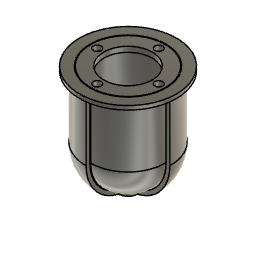
duba alt 2 v2 (Autodesk Fusion 360 design; units mm, degrees)
Autodesk Fusion 360 part; units mm, degrees
sketch "Eskiz1" plane through (0, 0, 0) normal (1, 0, 0) x (0, 1, 0)
  line L0 (-18.5, 0) -> (-28.5, 0)
  line L1 (-18.5, 0) -> (-18.5, -4)
  line L2 (-18.5, -4) -> (-28.5, -4)
  line L3 (-28.5, -4) -> (-28.5, 0)
  line L4 (-28.5, -4) -> (-25.5, -4)
  line L5 (-25.5, -4) -> (-25.5, -50)
  line L6 (-25.5, -50) -> (-28.5, -50)
  line L7 (-28.5, -50) -> (-28.5, -4)
  arc A0 (-28.5, -50) -> (-3.5325, -78.2802) centre (0, -50) ccw
  line L8 (-3.5325, -73.2631) -> (-3.5325, -72.7631)
  line L9 (-3.5325, -72.7631) -> (0, -72.7631)
  line L10 (-3.5325, -73.2631) -> (-3.5325, -75.2541)
  line L11 (-3.5325, -72.7631) -> (-5.5325, -72.7631)
  line L12 (-5.5325, -72.7631) -> (-5.5325, -74.8926)
  line L13 (-5.5325, -72.7631) -> (-5.5325, -70.7631)
  line L14 (-5.5325, -70.7631) -> (0, -70.7631)
  line L15 (0, -72.7631) -> (0, -70.7631)
  arc A1 (-25.5, -50) -> (-5.5325, -74.8926) centre (0, -50) ccw
  line L16 (-3.5325, -75.2541) -> (-3.5325, -78.2802)
  dimension "d2" = 10
  dimension "d3" = 2
  dimension "d4" = 2
  constraint perpendicular L0 L1
  constraint perpendicular L1 L2
  constraint coincident L2 L4.end
  constraint perpendicular L0 L5
  constraint perpendicular L5 L6
  constraint concentric A0 A1
  constraint tangent L5 A1
  constraint perpendicular L8 L9
  constraint coincident L10.end A1
  constraint perpendicular L9 L10
  constraint perpendicular L8 L11
  constraint perpendicular L11 L12
  constraint perpendicular L11 L13
  constraint perpendicular L14 L15
  constraint parallel L10 L16
  measures "d2" distance of L0.start L0.end
  measures "d3" distance of L8.end L11.end
  measures "d4" distance of L11.end L13.end
revolve "Döndür1" add sketch "Eskiz1" angle 110 about axis through (0, 0, 1.75) along (0, 0, 1) makes body 1
pattern_circular "C-Desen1" count 2 over 360 about axis through (0, 0, 1.75) along (0, 0, 1) of bodies 1 makes body 2
sketch "Eskiz2" plane through (0, 0, 0) normal (1, 0, 0) x (0, 1, 0)
  line L0 (3.5325, -72.7631) -> (3.5325, -78.2802)
  arc A0 (3.5325, -78.2802) -> (28.5, -50) centre (0, -50) ccw
  line L1 (28.5, -50) -> (28.5, -4)
  line L2 (28.5, -4) -> (28.5, 0)
  line L3 (28.5, 0) -> (18.5, 0)
  line L4 (18.5, 0) -> (18.5, -4)
  line L5 (18.5, -4) -> (25.5, -4)
  line L6 (25.5, -4) -> (25.5, -50)
  arc A1 (5.5325, -74.8926) -> (25.5, -50) centre (0, -50) ccw
  line L7 (5.5325, -74.8926) -> (5.5325, -70.7631)
  line L8 (5.5325, -70.7631) -> (0, -70.7631)
  line L9 (0, -70.7631) -> (0, -72.7631)
  line L10 (0, -72.7631) -> (3.5325, -72.7631)
  line L11 (5.5325, -74.8926) -> (5.5325, -77.9578)
  constraint coincident A1.start L7.start
  constraint coincident A0 L11.end
  constraint parallel L7 L11
revolve "Döndür2" add sketch "Eskiz2" angle 360 about axis through (0, 0, 1.75) along (0, 0, 1) contours L0 A0 L7 L8 L9 L10 L11 bodies 1 2
sketch "Eskiz3" plane through (0, 0, 0) normal (1, 0, 0) x (0, 1, 0)
  line L0 (5.5325, -74.8926) -> (5.5325, -77.9578)
  arc A0 (5.5325, -77.9578) -> (28.5, -50) centre (0, -50) ccw
  line L1 (28.5, -50) -> (28.5, -4)
  line L2 (28.5, -4) -> (28.5, 0)
  line L3 (28.5, 0) -> (18.5, 0)
  line L4 (18.5, 0) -> (18.5, -4)
  line L5 (18.5, -4) -> (25.5, -4)
  line L6 (25.5, -4) -> (25.5, -50)
  arc A1 (5.5325, -74.8926) -> (25.5, -50) centre (0, -50) ccw
  line L7 (18.5, 0) -> (28.5, 0)
  line L8 (28.5, 0) -> (28.5, -4)
  line L9 (28.5, -4) -> (18.5, -4)
  line L10 (18.5, -4) -> (18.5, 0)
  constraint horizontal L7
  constraint vertical L8
  constraint horizontal L9
  constraint vertical L10
  constraint coincident L1.end L2.start
  constraint coincident L3.end L4.start
revolve "Döndür3" add sketch "Eskiz3" angle 360 about axis through (0, 0, 1.75) along (0, 0, 1) contours L2 L3 L4 L5 L7 L8 L9 L10 bodies 1
sketch "Eskiz4" plane through (0, 0, 0) normal (0, 0, 1) x (-1, 0, 0)
  circle A0 centre (0, 0) radius 18.5
  circle A1 centre (0, 0) radius 28.5
  circle A2 centre (0, 23.5) radius 3
  circle A3 centre (-23.5, 0) radius 3
  circle A4 centre (0, -23.5) radius 3
  circle A5 centre (23.5, 0) radius 3
  dimension "d12" = 6
  dimension "d14" = 360
  measures "d12" diameter of A2
extrude "Ekstrüde Et1" cut sketch "Eskiz4" against normal blind 4 contours A2 | A3 | A4 | A5 bodies 1
sketch "Eskiz5" plane through (0, 0, 0) normal (0, 1, 0) x (1, 0, 0)
  line L0 (29, 0) -> (32, 0)
  line L1 (32, 3) -> (32, 50)
  line L2 (29, 50) -> (29, 0)
  line L3 (0, 82) -> (0, 79)
  arc A0 (32, 50) -> (0, 82) centre (0, 50) ccw
  arc A1 (29, 50) -> (0, 79) centre (0, 50) ccw
  line L4 (32, 0) -> (37, 0)
  line L5 (37, 0) -> (37, 3)
  line L6 (37, 3) -> (32, 3)
  constraint perpendicular L0 L1
  constraint concentric A0 A1
  constraint vertical L3
  constraint horizontal L4
  constraint vertical L5
  constraint horizontal L6
revolve "Döndür4" add sketch "Eskiz5" angle 90 about axis through (0, 0, -82) along (0, 0, 1) separate body makes body 3
pattern_circular "C-Desen2" count 2 over 360 about axis through (0, 0, -82) along (0, 0, 1) of bodies 3 makes body 4
sketch "Eskiz6" plane through (0, 0, 0) normal (-1, 0, 0) x (0, -1, 0)
  line L0 (-29, -50) -> (-29, 0)
  line L1 (-29, 0) -> (-37, 0)
  line L2 (-37, 0) -> (-37, -3)
  line L3 (-37, -3) -> (-32, -3)
  line L4 (-32, -3) -> (-32, -50)
  arc A0 (-32, -50) -> (0, -82) centre (0, -50) ccw
  line L5 (0, -82) -> (0, -79)
  arc A1 (-29, -50) -> (0, -79) centre (0, -50) ccw
  line L6 (0, -79.7) -> (-3, -79.7)
  line L7 (-3, -79.7) -> (-3, -78.5)
  line L8 (-3, -78.5) -> (-3, -78.3)
  line L9 (-3, -78.3) -> (-3, -73.3)
  line L10 (-3, -73.3) -> (0, -73.3)
  line L11 (0, -73.3) -> (0, -79.7)
  dimension "d20" = 5
  constraint coincident L5 L6.start
  constraint perpendicular L5 L6
  constraint perpendicular L6 L7
  constraint parallel L7 L8
  constraint parallel L8 L9
  constraint perpendicular L9 L10
  constraint perpendicular L6 L11
  measures "d20" distance of L8.end L9.end
revolve "Döndür5" add sketch "Eskiz6" angle 360 about axis through (0, 0, -73.3) along (0, 0, -1) contours A1 L7 L8 L9 L10 L11 bodies 3 4
sketch "Eskiz7" plane through (0, 0, 0) normal (0, 1, 0) x (-1, 0, 0)
  line L0 (29, 0) -> (29, -50)
  arc A0 (3, -78.8444) -> (29, -50) centre (0, -50) ccw
  arc A1 (0, -79) -> (3, -78.8444) centre (0, -50) ccw
  line L1 (0, -79) -> (0, -82)
  arc A2 (0, -82) -> (32, -50) centre (0, -50) ccw
  line L2 (32, -50) -> (32, -3)
  line L3 (32, -3) -> (37, -3)
  line L4 (37, -3) -> (37, 0)
  line L5 (37, 0) -> (29, 0)
  line L6 (29, 0) -> (37, 0)
  line L7 (37, 0) -> (37, -3)
  line L8 (37, -3) -> (29, -3)
  line L9 (29, -3) -> (29, 0)
  constraint horizontal L6
  constraint vertical L7
  constraint horizontal L8
  constraint vertical L9
  constraint coincident L3.end L4.start
  constraint coincident L0.start L5.end
revolve "Döndür6" add sketch "Eskiz7" angle 360 about axis through (0, 0, 1.75) along (0, 0, 1) contours L0 L3 L4 L5 L6 L7 L8 L9 bodies 3
sketch "Eskiz8" plane through (0, 0, 0) normal (0, 1, 0) x (-1, 0, 0)
  line L0 (32, -3) -> (29, -3)
  line L1 (29, -3) -> (29, -50)
  arc A0 (3, -78.8444) -> (29, -50) centre (0, -50) ccw
  arc A1 (0, -79) -> (3, -78.8444) centre (0, -50) ccw
  line L2 (0, -79) -> (0, -82)
  arc A2 (0, -82) -> (32, -50) centre (0, -50) ccw
  line L3 (32, -50) -> (32, -3)
  line L4 (6.5435, -78.2521) -> (7.1205, -81.1977)
  constraint coincident A0 L4.start
  constraint coincident A2 L4.end
revolve "Döndür7" add sketch "Eskiz8" angle 360 about axis through (0, 0, 1.75) along (0, 0, 1) contours A0 A1 L2 A2 L4 bodies 3
